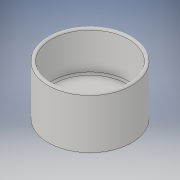
# Autodesk Inventor part: 30-30-RearSight
Saved by Autodesk Inventor 2019.2 (Build 232265000, 265)
## iProperties
Created: 2018-10-16
Part Number: 30-30-RearSight
Material: Generic
Document SubType Name: Modeling
Designer: steele
Density: 1 g/cm^3
Appearance: Default
Author: steele
Autodesk Inventor part; units mm, degrees
ref_plane "YZ Plane" through (0, 0, 0) normal (1, 0, 0) x (0, 1, 0)
ref_plane "XZ Plane" through (0, 0, 0) normal (0, 1, 0) x (-1, 0, 0)
ref_plane "XY Plane" through (0, 0, 0) normal (0, 0, 1) x (1, 0, 0)
sketch "Sketch1" plane through (0, 0, 0) normal (0, 1, 0) x (-1, 0, 0)
  circle A0 centre (0, 0) radius 20.1295
  dimension "d0" = 40.259
  constraints: 1 centre point, 1 coincident
  measures "d0" diameter of A0
extrude "Extrusion1" add sketch "Sketch1" against normal blind 6.35
sketch "Sketch2" plane through (0, 0, 0) normal (0, 1, 0) x (1, 0, 0)
  circle A0 centre (0, 0) radius 20.1295
  circle A1 centre (0, 0) radius 18.542
  dimension "d3" = 37.084
  dimension "d4" = 40.259
  constraints: 2 centre point, 2 coincident
  measures "d3" diameter of A1
  measures "d4" diameter of A0
extrude "Extrusion2" add sketch "Sketch2" along normal blind 19.05
sketch "Sketch3" plane through (0, -6.35, 0) normal (0, -1, 0) x (1, 0, 0)
  circle A0 centre (0, 0) radius 20.1295 construction
  line L0 (20.1295, 0) -> (-20.1295, 0) construction
  line L1 (13.6024, 3.048) -> (16.8826, 3.048)
  line L2 (16.8826, 3.048) -> (16.8826, 1.9859)
  line L3 (16.8826, 1.9859) -> (16.0082, 1.9859)
  line L4 (16.0082, 1.9859) -> (16.0082, -1.9859)
  line L5 (16.0082, -1.9859) -> (16.8826, -1.9859)
  line L6 (16.8826, -1.9859) -> (16.8826, -3.048)
  line L7 (16.8826, -3.048) -> (13.6024, -3.048)
  line L8 (13.6024, -3.048) -> (13.6024, -1.9859)
  line L9 (13.6024, -1.9859) -> (14.4768, -1.9859)
  line L10 (14.4768, -1.9859) -> (14.4768, 1.9859)
  line L11 (14.4768, 1.9859) -> (13.6024, 1.9859)
  line L12 (13.6024, 1.9859) -> (13.6024, 3.048)
  spline S0 degree 2 poles (7.1458, 0.0049) (7.1458, 0.8596) (7.8917, 2.2033) (8.4598, 2.5639) knots 0 0 0 1 2 2 2
  spline S1 degree 2 poles (8.4598, 2.5639) (8.934, 2.8702) (10.0505, 3.048) (10.6779, 3.048) knots 0 0 0 1 2 2 2
  line L13 (10.6779, 3.048) -> (12.5847, 3.048)
  line L14 (12.5847, 3.048) -> (12.5847, -3.048)
  line L15 (12.5847, -3.048) -> (10.6976, -3.048)
  spline S2 degree 2 poles (10.6976, -3.048) (10.0554, -3.048) (8.934, -2.885) (8.44, -2.5688) knots 0 0 0 1 2 2 2
  spline S3 degree 2 poles (8.44, -2.5688) (7.8423, -2.1835) (7.1458, -0.8793) (7.1458, 0.0049) knots 0 0 0 1 2 2 2
  spline S4 degree 2 poles (8.7167, -0.0049) (8.7167, -0.6076) (9.1316, -1.4672) (9.5565, -1.7093) knots 0 0 0 1 2 2 2
  spline S5 degree 2 poles (9.5565, -1.7093) (9.8677, -1.8772) (10.5494, -1.9118) (11.0237, -1.9118) knots 0 0 0 1 2 2 2
  line L16 (11.0237, -1.9118) -> (11.0533, -1.9118)
  line L17 (11.0533, -1.9118) -> (11.0533, 1.9069)
  line L18 (11.0533, 1.9069) -> (11.0237, 1.9069)
  spline S6 degree 2 poles (11.0237, 1.9069) (10.5099, 1.9069) (9.8035, 1.8723) (9.4824, 1.6697) knots 0 0 0 1 2 2 2
  spline S7 degree 2 poles (9.4824, 1.6697) (9.1069, 1.4326) (8.7167, 0.5977) (8.7167, -0.0049) knots 0 0 0 1 2 2 2
  line L19 (4.6214, 0.0593) -> (6.0688, 0.0593)
  line L20 (6.0688, 0.0593) -> (6.0688, -1.5512)
  line L21 (6.0688, -1.5512) -> (4.6214, -1.5512)
  line L22 (4.6214, -1.5512) -> (4.6214, 0.0593)
  line L23 (4.6214, 3.048) -> (6.0688, 3.048)
  line L24 (6.0688, 3.048) -> (6.0688, 1.4375)
  line L25 (6.0688, 1.4375) -> (4.6214, 1.4375)
  line L26 (4.6214, 1.4375) -> (4.6214, 3.048)
  line L27 (-3.4556, 3.048) -> (0.5706, 3.048)
  line L28 (0.5706, 3.048) -> (0.5706, 1.9859)
  line L29 (0.5706, 1.9859) -> (-0.7138, 1.9859)
  line L30 (-0.7138, 1.9859) -> (-0.7138, -1.2399)
  line L31 (-0.7138, -1.2399) -> (0.5706, -1.2399)
  line L32 (0.5706, -1.2399) -> (0.5706, -2.2329)
  spline S8 degree 2 poles (0.5706, -2.2329) (0.289, -2.2329) (-0.2692, -2.307) (-0.4372, -2.386) knots 0 0 0 1 2 2 2
  spline S9 degree 2 poles (-0.4372, -2.386) (-0.6299, -2.4848) (-0.8472, -2.8158) (-0.867, -3.0628) knots 0 0 0 1 2 2 2
  line L33 (-0.867, -3.0628) -> (-2.2008, -3.0628)
  line L34 (-2.2008, -3.0628) -> (-2.2008, 1.9859)
  line L35 (-2.2008, 1.9859) -> (-3.4556, 1.9859)
  line L36 (-3.4556, 1.9859) -> (-3.4556, 3.048)
  line L37 (-5.9997, 3.048) -> (-4.5522, 3.048)
  line L38 (-4.5522, 3.048) -> (-4.5522, 1.4375)
  line L39 (-4.5522, 1.4375) -> (-5.9997, 1.4375)
  line L40 (-5.9997, 1.4375) -> (-5.9997, 3.048)
  line L41 (-11.7597, 1.6253) -> (-10.9348, 1.6253)
  line L42 (-10.9348, 1.6253) -> (-10.9348, 3.0628)
  line L43 (-10.9348, 3.0628) -> (-9.4577, 3.0628)
  line L44 (-9.4577, 3.0628) -> (-9.4577, 1.6253)
  line L45 (-9.4577, 1.6253) -> (-6.7703, 1.6253)
  line L46 (-6.7703, 1.6253) -> (-6.7703, 0.4891)
  line L47 (-6.7703, 0.4891) -> (-9.4083, -3.048)
  line L48 (-9.4083, -3.048) -> (-10.9348, -3.048)
  line L49 (-10.9348, -3.048) -> (-10.9348, 0.5286)
  line L50 (-10.9348, 0.5286) -> (-11.7597, 0.5286)
  line L51 (-11.7597, 0.5286) -> (-11.7597, 1.6253)
  line L52 (-9.4577, 0.5286) -> (-9.4577, -1.5462)
  line L53 (-9.4577, -1.5462) -> (-7.9115, 0.5286)
  line L54 (-7.9115, 0.5286) -> (-9.4577, 0.5286)
  spline S10 degree 2 poles (-16.9912, 0.9732) (-16.9912, 1.9365) (-15.7711, 3.1764) (-14.704, 3.1764) knots 0 0 0 1 2 2 2
  spline S11 degree 2 poles (-14.704, 3.1764) (-14.1705, 3.1764) (-13.3356, 2.8702) (-13.0442, 2.5688) knots 0 0 0 1 2 2 2
  spline S12 degree 2 poles (-13.0442, 2.5688) (-12.6984, 2.2181) (-12.3279, 1.1066) (-12.3279, 0.331) knots 0 0 0 1 2 2 2
  spline S13 degree 2 poles (-12.3279, 0.331) (-12.3279, -0.4693) (-12.6737, -1.7142) (-13.0639, -2.1934) knots 0 0 0 1 2 2 2
  spline S14 degree 2 poles (-13.0639, -2.1934) (-13.4344, -2.6479) (-14.6398, -3.1616) (-15.4648, -3.1616) knots 0 0 0 1 2 2 2
  spline S15 degree 2 poles (-15.4648, -3.1616) (-15.7661, -3.1616) (-16.3688, -3.0826) (-16.4775, -3.0579) knots 0 0 0 1 2 2 2
  line L55 (-16.4775, -3.0579) -> (-16.4775, -1.8624)
  line L56 (-16.4775, -1.8624) -> (-16.3688, -1.8624)
  spline S16 degree 2 poles (-16.3688, -1.8624) (-16.2601, -1.9167) (-15.7661, -2.0501) (-15.45, -2.0501) knots 0 0 0 1 2 2 2
  spline S17 degree 2 poles (-15.45, -2.0501) (-14.7336, -2.0501) (-13.9531, -1.2943) (-13.8593, -0.5928) knots 0 0 0 1 2 2 2
  spline S18 degree 2 poles (-13.8593, -0.5928) (-14.1606, -0.7855) (-14.7781, -1.0127) (-15.1684, -1.0127) knots 0 0 0 1 2 2 2
  spline S19 degree 2 poles (-15.1684, -1.0127) (-15.4994, -1.0127) (-16.0773, -0.8349) (-16.2996, -0.6669) knots 0 0 0 1 2 2 2
  spline S20 degree 2 poles (-16.2996, -0.6669) (-16.6158, -0.4248) (-16.9912, 0.3606) (-16.9912, 0.9732) knots 0 0 0 1 2 2 2
  spline S21 degree 2 poles (-15.2079, 1.892) (-15.3265, 1.7438) (-15.4549, 1.398) (-15.4549, 1.0473) knots 0 0 0 1 2 2 2
  spline S22 degree 2 poles (-15.4549, 1.0473) (-15.4549, 0.7509) (-15.3067, 0.3656) (-15.1733, 0.2519) knots 0 0 0 1 2 2 2
  spline S23 degree 2 poles (-15.1733, 0.2519) (-15.035, 0.1334) (-14.6941, 0.0494) (-14.5015, 0.0494) knots 0 0 0 1 2 2 2
  spline S24 degree 2 poles (-14.5015, 0.0494) (-14.3384, 0.0494) (-14.0025, 0.1334) (-13.8543, 0.1927) knots 0 0 0 1 2 2 2
  spline S25 degree 2 poles (-13.8543, 0.1927) (-13.8543, 0.2322) (-13.8444, 0.4199) (-13.8444, 0.5632) knots 0 0 0 1 2 2 2
  spline S26 degree 2 poles (-13.8444, 0.5632) (-13.8444, 1.0917) (-14.0272, 1.729) (-14.1705, 1.892) knots 0 0 0 1 2 2 2
  spline S27 degree 2 poles (-14.1705, 1.892) (-14.2742, 2.0254) (-14.5509, 2.139) (-14.6991, 2.139) knots 0 0 0 1 2 2 2
  spline S28 degree 2 poles (-14.6991, 2.139) (-14.8226, 2.139) (-15.1091, 2.0155) (-15.2079, 1.892) knots 0 0 0 1 2 2 2
  constraints: 2 end point, 2 horizontal, 2 point on circle
extrude "Extrusion3" cut sketch "Sketch3" against normal blind 3.175
fillet "Fillet2" radius 0.7937 4 edges at (-20.1295, 19.05, 0) (-18.542, 19.05, 0) (-18.542, 0, 0) (20.1295, -6.35, 0)
equation "\"d0\" = outerDiam"
equation "\"d1\" = endCapThickness"
equation "\"d3\" = internalDiam"
equation "\"d4\" = outerDiam"
equation "\"d5\" = length"
equation "\"length\" = 19.05"
equation "\"internalDiam\" = 37.084"
equation "\"wallThickness\" = 1.5875"
equation "\"endCapThickness\" = 6.35"
equation "\"outerDiam\" = internalDiam + 2 * wallThickness"
body "Solid1"
